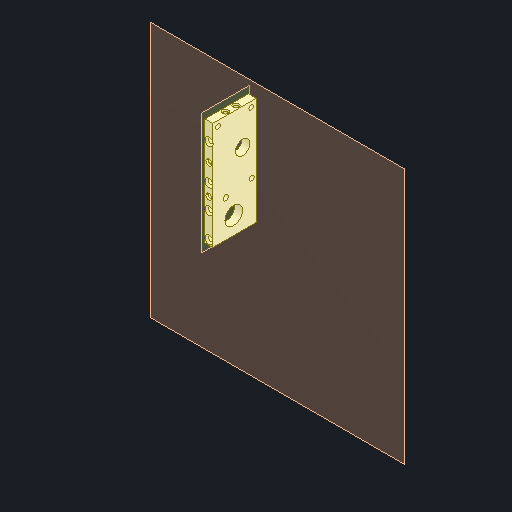
# Autodesk Inventor part: right_gear_holder
Saved by Autodesk Inventor 2023 (Build 270158000, 158)
## iProperties
Created: 2024-04-23
Part Number: right_gear_holder
Material: Nylon 6/6
Document SubType Name: Modeling
Designer: szymo
Density: 1.13 g/cm^3
Appearance: Nylon 6
Mass: 14.9327 g
Surface Area: 88.4291 cm^2
Volume: 13.2148 cm^3
Author: szymo
Autodesk Inventor part; units mm, degrees
ref_plane "YZ Plane" through (0, 0, 0) normal (1, 0, 0) x (0, 1, 0)
ref_plane "XZ Plane" through (0, 0, 0) normal (0, 1, 0) x (-1, 0, 0)
ref_plane "Work Plane1" through (0, 0, 0) normal (0, 0, 1) x (1, 0, 0)
sketch "Sketch1" plane through (0, 0, 0) normal (0, 0, 1) x (1, 0, 0)
  line L0 (23.5, 88.5) -> (-23.5, 88.5) projected
  line L1 (-23.5, 88.5) -> (-23.5, 36.5) projected
  line L2 (-26.5, 33.5) -> (-89, 33.5) projected
  line L3 (-89, 33.5) -> (-89, -72.5) projected
  line L4 (-89, -72.5) -> (-77, -72.5) projected
  line L5 (-74, -75.5) -> (-74, -93.5) projected
  line L6 (-74, -93.5) -> (74, -93.5) projected
  line L7 (74, -93.5) -> (74, -75.5) projected
  line L8 (77, -72.5) -> (89, -72.5) projected
  line L9 (89, -72.5) -> (89, 33.5) projected
  line L10 (89, 33.5) -> (26.5, 33.5) projected
  line L11 (23.5, 36.5) -> (23.5, 88.5) projected
  line L12 (-4.5, 81.5) -> (-4.5, 36.5) projected
  line L13 (-7.5, 33.5) -> (-13.5, 33.5) projected
  line L14 (-16.5, 36.5) -> (-16.5, 81.5) projected
  line L15 (7.5, 84.5) -> (13.5, 84.5) projected
  line L16 (16.5, 81.5) -> (16.5, 36.5) projected
  line L17 (13.5, 33.5) -> (7.5, 33.5) projected
  line L18 (4.5, 36.5) -> (4.5, 81.5) projected
  line L19 (-13.5, 84.5) -> (-7.5, 84.5) projected
  line L20 (-16.5, 88.5) -> (-22.5, 88.5)
  line L21 (-22.5, 88.5) -> (-22.5, 3.75)
  line L22 (-22.5, 3.75) -> (-16.5, 3.75)
  line L23 (-16.5, 3.75) -> (-16.5, 88.5)
  line L24 (-32.2, 4.75) -> (-59.9, 4.75)
  arc A0 (13.5, 33.5) -> (16.5, 36.5) centre (13.5, 36.5) ccw projected
  arc A1 (4.5, 36.5) -> (7.5, 33.5) centre (7.5, 36.5) ccw projected
  arc A2 (7.5, 84.5) -> (4.5, 81.5) centre (7.5, 81.5) ccw projected
  arc A3 (16.5, 81.5) -> (13.5, 84.5) centre (13.5, 81.5) ccw projected
  arc A4 (-4.5, 81.5) -> (-7.5, 84.5) centre (-7.5, 81.5) ccw projected
  arc A5 (-7.5, 33.5) -> (-4.5, 36.5) centre (-7.5, 36.5) ccw projected
  arc A6 (-16.5, 36.5) -> (-13.5, 33.5) centre (-13.5, 36.5) ccw projected
  arc A7 (-13.5, 84.5) -> (-16.5, 81.5) centre (-13.5, 81.5) ccw projected
  arc A8 (-26.5, 33.5) -> (-23.5, 36.5) centre (-26.5, 36.5) ccw projected
  arc A9 (-74, -75.5) -> (-77, -72.5) centre (-77, -75.5) ccw projected
  arc A10 (77, -72.5) -> (74, -75.5) centre (77, -75.5) ccw projected
  arc A11 (23.5, 36.5) -> (26.5, 33.5) centre (26.5, 36.5) ccw projected
  circle A12 centre (39.125, 25.9125) radius 1.0065 projected
  circle A13 centre (72.95, 12.275) radius 1.0065 projected
  circle A14 centre (-39.125, 12.3375) radius 1.0065 projected
  circle A15 centre (-72.95, 25.975) radius 1.0065 projected
  circle A16 centre (-72.95, 12.275) radius 1.0065 projected
  circle A17 centre (-39.125, 25.9125) radius 1.0065 projected
  circle A18 centre (72.95, 25.975) radius 1.0065 projected
  circle A19 centre (39.125, 12.3375) radius 1.0065 projected
  circle A20 centre (-42.4984, -44.6666) radius 1.2295 projected
  circle A21 centre (-79, -42.3889) radius 1.2295 projected
  circle A22 centre (-19.5, 28.875) radius 1.2295 projected
  circle A23 centre (19.5, 9.55) radius 1.2295 projected
  circle A24 centre (19.5, 47.3) radius 1.2295 projected
  circle A25 centre (-19.5, 47.3) radius 1.2295 projected
  circle A26 centre (0, 74.7) radius 1.2295 projected
  circle A27 centre (-19.4231, 74.8077) radius 1.2295 projected
  circle A28 centre (19.5, 74.7) radius 1.2295 projected
  circle A29 centre (0, 49.05) radius 1.2295 projected
  circle A30 centre (19.5, 28.875) radius 1.2295 projected
  circle A31 centre (0, 19.125) radius 1.2295 projected
  circle A32 centre (-19.5, 9.55) radius 1.2295 projected
  circle A33 centre (42.5, -44.6649) radius 1.2295 projected
  circle A34 centre (79, -42.3889) radius 1.2295 projected
  circle A35 centre (21.5, -85.5) radius 1.8 projected
  circle A36 centre (-64.5, -85.5) radius 1.8 projected
  circle A37 centre (-21.5, -85.5) radius 1.8 projected
  circle A38 centre (64.5, -85.5) radius 1.8 projected
  line L25 (-57, -78.5) -> (-82, -60.2553) projected
  line L26 (-82, -60.2553) -> (-82, -45.3889) projected
  line L27 (-76, -45.3889) -> (-45.4984, -47.6666) projected
  line L28 (-21.1, -27.9) -> (-21.1, -21.9) projected
  line L29 (-45.4984, -41.6666) -> (-76, -39.3889) projected
  line L30 (-82, -39.3889) -> (-82, 4.75) projected
  line L31 (30.3333, 4.75) -> (82, 4.75) projected
  line L32 (82, 4.75) -> (82, -39.3889) projected
  line L33 (76, -39.3889) -> (45.5, -41.6649) projected
  line L34 (21.1, -21.9) -> (21.1, -27.9) projected
  line L35 (45.5, -47.6649) -> (76, -45.3889) projected
  line L36 (82, -45.3889) -> (82, -60.2553) projected
  line L37 (82, -60.2553) -> (57, -78.5) projected
  line L38 (57, -78.5) -> (57, -87.5) projected
  arc A39 (55, -89.5) -> (57, -87.5) centre (55, -87.5) ccw projected
  line L39 (55, -89.5) -> (31, -89.5) projected
  arc A40 (29, -87.5) -> (31, -89.5) centre (31, -87.5) ccw projected
  line L40 (29, -87.5) -> (29, -78.5) projected
  line L41 (14, -78.5) -> (14, -87.5) projected
  arc A41 (12, -89.5) -> (14, -87.5) centre (12, -87.5) ccw projected
  line L42 (12, -89.5) -> (-12, -89.5) projected
  arc A42 (-14, -87.5) -> (-12, -89.5) centre (-12, -87.5) ccw projected
  line L43 (-14, -87.5) -> (-14, -78.5) projected
  line L44 (-29, -78.5) -> (-29, -87.5) projected
  arc A43 (-31, -89.5) -> (-29, -87.5) centre (-31, -87.5) ccw projected
  line L45 (-31, -89.5) -> (-55, -89.5) projected
  arc A44 (-57, -87.5) -> (-55, -89.5) centre (-55, -87.5) ccw projected
  line L46 (-57, -87.5) -> (-57, -78.5) projected
  line L47 (-69.95, 28.9125) -> (-42.125, 28.9125) projected
  line L48 (-42.125, 28.9125) -> (-42.125, 9.275) projected
  line L49 (-42.125, 9.275) -> (-69.95, 9.275) projected
  line L50 (-69.95, 9.275) -> (-69.95, 28.9125) projected
  line L51 (-16.5, 9.75) -> (-16.5, 28.5) projected
  line L52 (-16.5, 28.5) -> (-4.5, 28.5) projected
  line L53 (-4.5, 28.5) -> (-4.5, 9.75) projected
  line L54 (-4.5, 9.75) -> (-16.5, 9.75) projected
  line L55 (69.95, 9.3375) -> (42.125, 9.3375) projected
  line L56 (42.125, 9.3375) -> (42.125, 28.975) projected
  line L57 (42.125, 28.975) -> (69.95, 28.975) projected
  line L58 (69.95, 28.975) -> (69.95, 9.3375) projected
  line L59 (4.5, 9.75) -> (4.5, 28.5) projected
  line L60 (4.5, 28.5) -> (16.5, 28.5) projected
  line L61 (16.5, 28.5) -> (16.5, 9.75) projected
  line L62 (16.5, 9.75) -> (4.5, 9.75) projected
  line L63 (45.5, -41.6649) -> (27.1, -21.9) projected
  line L64 (27.1, -21.9) -> (30.3333, 4.75) projected
  line L65 (-45.4984, -47.6666) -> (-29, -78.5) projected
  line L66 (-82, 4.75) -> (-30.3333, 4.75) projected
  line L67 (-30.3333, 4.75) -> (-27.1, -21.9) projected
  line L68 (-27.1, -21.9) -> (-45.4984, -41.6666) projected
  line L69 (29, -78.5) -> (45.5, -47.6649) projected
  line L70 (-14, -78.5) -> (-39, -45.3279) projected
  line L71 (-39, -44.2124) -> (-21.1, -27.9) projected
  line L72 (-21.1, -21.9) -> (-24.3333, 4.75) projected
  line L73 (-24.3333, 4.75) -> (24.3333, 4.75) projected
  line L74 (24.3333, 4.75) -> (21.1, -21.9) projected
  line L75 (21.1, -27.9) -> (39.5, -44.6649) projected
  line L76 (39.5, -44.6649) -> (14, -78.5) projected
  circle A45 centre (-78, -67.1725) radius 1.2295 projected
  circle A46 centre (78, -67.1725) radius 1.2295 projected
  line L77 (-22.5, 28.9125) -> (-22.5, 9.55) projected
  line L78 (-22.5, 9.55) -> (-36.125, 9.55) projected
  line L79 (-36.125, 9.55) -> (-36.125, 28.9125) projected
  line L80 (-36.125, 28.9125) -> (-22.5, 28.9125) projected
  line L81 (76, -45.3889) -> (82, -45.3889) projected
  line L82 (82, -39.3889) -> (76, -39.3889) projected
  line L83 (36.125, 9.275) -> (22.5, 9.275) projected
  line L84 (22.5, 9.275) -> (22.5, 28.9125) projected
  line L85 (22.5, 28.9125) -> (36.125, 28.9125) projected
  line L86 (36.125, 28.9125) -> (36.125, 9.275) projected
  line L87 (-86, 28.975) -> (-75.95, 28.975) projected
  line L88 (-75.95, 28.975) -> (-75.95, 9.275) projected
  line L89 (-75.95, 9.275) -> (-86, 9.275) projected
  line L90 (-86, 9.275) -> (-86, 28.975) projected
  line L91 (-82, -45.3889) -> (-76, -45.3889) projected
  line L92 (-76, -39.3889) -> (-82, -39.3889) projected
  line L93 (75.95, 28.975) -> (86, 28.975) projected
  line L94 (86, 28.975) -> (86, 9.275) projected
  line L95 (86, 9.275) -> (75.95, 9.275) projected
  line L96 (75.95, 9.275) -> (75.95, 28.975) projected
  line L97 (-39, -45.3279) -> (-39, -44.2124) projected
  circle A47 centre (-24.1, -73.1) radius 1.2295 projected
  circle A48 centre (24.1, -24.9) radius 1.2295 projected
  circle A49 centre (-24.1, -24.9) radius 1.2295 projected
  circle A50 centre (24.1, -73.1) radius 1.2295 projected
  point P0 (0, 0)
  point P1 (-16.5, 36.5)
  point P2 (-16.5, 81.5)
  point P3 (7.5, 81.5)
  point P4 (13.5, 81.5)
  point P5 (-7.5, 81.5)
  point P6 (-13.5, 81.5)
  point P7 (-77, -75.5)
  point P8 (39, -44.2094)
  point P9 (-79, -67.8878)
  point P10 (-79, -66.4572)
  point P11 (-22.5, 25.9125)
  point P12 (-22.5, 12.55)
  point P13 (7.5, 81.5)
  point P14 (13.5, 81.5)
  point P15 (-7.5, 81.5)
  point P16 (-13.5, 81.5)
  dimension "d0" = 1
  dimension "d2" = 1
  constraints: 10 end point, 2 horizontal, 2 parallel, 1 collinear, 1 perpendicular, 1 point on line, 2 other
  measures "d0" distance between parallel lines of L1 L21
  measures "d2" distance between parallel lines of L24 L22
ref_plane "Work Plane2" through (-89, -40.3889, 33.5) normal (0, 0, 1) x (1, 0, 0)
extrude "Extrusion1" add sketch "Sketch1" along normal up to surface (33.5 mm away) contours L23 L14 L73 L21 L0 | L73 L23 L22 L21 | A22 | A25 | A27 | A32
sketch "Sketch2" plane through (-22.5, 3.75, 0) normal (-1, 0, 0) x (0, 0, 1)
  arc A0 (15.7043, 9.7757) -> (16.863, 11.545) centre (12.3771, 13.2188) ccw projected
  arc A1 (16.863, 11.545) -> (17.4685, 11.512) centre (17.375, 15.375) ccw projected
  arc A2 (17.4685, 11.512) -> (18.4285, 9.6275) centre (22.1095, 12.6893) ccw projected
  arc A3 (18.4285, 9.6275) -> (19.3146, 9.863) centre (17.375, 15.375) ccw projected
  arc A4 (19.3146, 9.863) -> (19.2121, 11.9755) centre (14.599, 10.6929) ccw projected
  arc A5 (19.2121, 11.9755) -> (19.7212, 12.3047) centre (17.375, 15.375) ccw projected
  arc A6 (19.7212, 12.3047) -> (21.6056, 11.3444) centre (22.7839, 15.9851) ccw projected
  arc A7 (21.6056, 11.3444) -> (22.184, 12.0558) centre (17.375, 15.375) ccw projected
  arc A8 (22.184, 12.0558) -> (20.8594, 13.7045) centre (17.8813, 9.9554) ccw projected
  arc A9 (20.8594, 13.7045) -> (21.0778, 14.2702) centre (17.375, 15.375) ccw projected
  arc A10 (21.0778, 14.2702) -> (23.1668, 14.6008) centre (21.3923, 19.0479) ccw projected
  arc A11 (23.1668, 14.6008) -> (23.2166, 15.5164) centre (17.375, 15.375) ccw projected
  arc A12 (23.2166, 15.5164) -> (21.1758, 16.0716) centre (20.9701, 11.288) ccw projected
  arc A13 (21.1758, 16.0716) -> (21.02, 16.6576) centre (17.375, 15.375) ccw projected
  arc A14 (21.02, 16.6576) -> (22.5157, 18.153) centre (18.4662, 20.7077) ccw projected
  arc A15 (22.5157, 18.153) -> (22.0178, 18.923) centre (17.375, 15.375) ccw projected
  arc A16 (22.0178, 18.923) -> (20.0404, 18.1726) centre (22.6858, 14.1817) ccw projected
  arc A17 (20.0404, 18.1726) -> (19.57, 18.5552) centre (17.375, 15.375) ccw projected
  arc A18 (19.57, 18.5552) -> (19.9011, 20.644) centre (15.1233, 20.3306) ccw projected
  arc A19 (19.9011, 20.644) -> (19.0457, 20.9743) centre (17.375, 15.375) ccw projected
  arc A20 (19.0457, 20.9743) -> (17.887, 19.205) centre (22.3729, 17.5312) ccw projected
  arc A21 (17.887, 19.205) -> (17.2815, 19.238) centre (17.375, 15.375) ccw projected
  arc A22 (17.2815, 19.238) -> (16.3215, 21.1225) centre (12.6405, 18.0607) ccw projected
  arc A23 (16.3215, 21.1225) -> (15.4354, 20.887) centre (17.375, 15.375) ccw projected
  arc A24 (15.4354, 20.887) -> (15.5379, 18.7745) centre (20.151, 20.0571) ccw projected
  arc A25 (15.5379, 18.7745) -> (15.0288, 18.4453) centre (17.375, 15.375) ccw projected
  arc A26 (15.0288, 18.4453) -> (13.1444, 19.4056) centre (11.9661, 14.7649) ccw projected
  arc A27 (13.1444, 19.4056) -> (12.566, 18.6942) centre (17.375, 15.375) ccw projected
  arc A28 (12.566, 18.6942) -> (13.8906, 17.0455) centre (16.8687, 20.7946) ccw projected
  arc A29 (13.8906, 17.0455) -> (13.6722, 16.4798) centre (17.375, 15.375) ccw projected
  arc A30 (13.6722, 16.4798) -> (11.5832, 16.1492) centre (13.3577, 11.7021) ccw projected
  arc A31 (11.5832, 16.1492) -> (11.5334, 15.2336) centre (17.375, 15.375) ccw projected
  arc A32 (11.5334, 15.2336) -> (13.5742, 14.6784) centre (13.7799, 19.462) ccw projected
  arc A33 (13.5742, 14.6784) -> (13.73, 14.0924) centre (17.375, 15.375) ccw projected
  arc A34 (13.73, 14.0924) -> (12.2343, 12.597) centre (16.2838, 10.0423) ccw projected
  arc A35 (12.2343, 12.597) -> (12.7322, 11.827) centre (17.375, 15.375) ccw projected
  arc A36 (12.7322, 11.827) -> (14.7096, 12.5774) centre (12.0642, 16.5683) ccw projected
  arc A37 (14.7096, 12.5774) -> (15.18, 12.1948) centre (17.375, 15.375) ccw projected
  arc A38 (15.18, 12.1948) -> (14.8489, 10.106) centre (19.6267, 10.4194) ccw projected
  arc A39 (14.8489, 10.106) -> (15.7043, 9.7757) centre (17.375, 15.375) ccw projected
  circle A40 centre (17.375, 15.375) radius 6.75
  circle A41 centre (17.375, 15.375) radius 5.8433
  line L0 (23.2183, 15.375) -> (24.125, 15.375)
  circle A42 centre (10.5, 57.25) radius 5.5 projected
  point P0 (0, -3.75)
  dimension "d6" = 13.5
  dimension "d5" = 0.9067
  dimension "d9" = 11
  constraints: 3 horizontal, 2 coincident, 2 end point, 2 horizontal alignment, 5 other
  measures "d5" distance of L0.start L0.end
  measures "d9" diameter of A42
extrude "Extrusion2" cut sketch "Sketch2" against normal up to next contours A39 A38 A37 A36 A35 A34 A33 A32 A31 A30 A29 A28 A27 A26 A25 A24 A23 A22 A21 A20 A19 A18 A17 A16 A15 A14 A13 A12 A11 A10 A9 A8 A7 A6 A5 A4 A3 A2 A1 A0 | A0 A1 A2 A41 | A41 A36 A37 A38 | A4 A5 A6 A41 | A41 A32 A33 A34 | A8 A9 A10 A41 | A41 A28 A29 A30 | A41 A24 A25 A26 | A12 A13 A14 A41 | A41 A20 A21 A22 | A16 A17 A18 A41 | A40 | A42
sketch "Sketch3" plane through (-16.5, 3.75, 0) normal (1, 0, 0) x (0, 0, -1)
  circle A0 centre (-23.4363, 30.1825) radius 2 projected
  point P0 (0, -3.75)
extrude "Extrusion3" cut sketch "Sketch3" against normal blind 5
ref_plane "Work Plane3" through (-23.5, 3.75, 0) normal (-1, 0, 0) x (0, 0, 1)
sketch "Sketch5" plane through (-23.5, 3.75, 0) normal (-1, 0, 0) x (0, 0, 1)
  circle A0 centre (29.5, 80.75) radius 2.1 projected
  circle A1 centre (4, 80.75) radius 2.1 projected
  circle A2 centre (3.5, 33.25) radius 2.1 projected
  point P0 (0, -3.75)
hole "Hole1" at (-23.5, 84.5, 29.5) at (-23.5, 84.5, 4) at (-23.5, 37, 3.5) direction (1, 0, 0) diameter 3.6 end through all countersink diameter 6.2 countersink angle 90 clearance for "Countersunk Flat Head Screw ISO 2009/7046" size "M3" standard "ISO"
sketch "Sketch6" plane through (-22.5, 3.75, 33.5) normal (0, 0, 1) x (1, 0, 0)
  line L0 (0, 8.625) -> (0, 22.125) projected
  line L1 (1, 32.1825) -> (1, 28.1825) projected
  line L2 (0, 31.15) -> (0, 35.35) projected
  line L3 (0, 51.75) -> (0, 62.75) projected
  line L4 (0, 78.65) -> (0, 82.85) projected
  line L5 (0, 78.65) -> (0, 82.85) projected
  line L6 (6, 0) -> (0, 0) projected
  line L7 (6, 84.75) -> (6, 0) projected
  line L8 (0, 84.75) -> (6, 84.75) projected
  line L9 (0, 0) -> (0, 84.75) projected
  line L10 (6, 28.125) -> (0, 28.125)
  line L11 (0, 28.125) -> (0, 35.35)
  line L12 (0, 35.35) -> (6, 35.35)
  line L13 (6, 35.35) -> (6, 28.125)
  line L14 (0, 8.625) -> (6, 8.625) projected
  line L15 (6, 8.625) -> (0, 8.625)
  line L16 (0, 8.625) -> (0, 22.125)
  line L17 (0, 22.125) -> (6, 22.125)
  line L18 (6, 22.125) -> (6, 8.625)
  line L19 (6, 78.95) -> (0.3, 78.95) projected
  line L20 (6, 84.75) -> (0, 84.75) projected
  line L21 (6, 78.95) -> (0, 78.95)
  line L22 (0, 78.95) -> (0, 84.75)
  line L23 (0, 84.75) -> (6, 84.75)
  line L24 (6, 84.75) -> (6, 78.95)
  line L25 (0, 51.75) -> (6, 51.75) projected
  line L26 (0, 51.75) -> (0, 62.75) projected
  line L27 (6, 51.75) -> (0, 51.75)
  line L28 (0, 51.75) -> (0, 62.75)
  line L29 (0, 62.75) -> (6, 62.75)
  line L30 (6, 62.75) -> (6, 51.75)
  line L31 (6, 0) -> (0, 0)
  line L32 (0, 0) -> (0, 4)
  line L33 (0, 4) -> (6, 4)
  line L34 (6, 4) -> (6, 0)
  circle A0 centre (3, 5.8) radius 1.8
  line L35 (6, 22.125) -> (0, 28.125)
  line L36 (0, 22.125) -> (6, 28.125)
  line L37 (6, 35.35) -> (0, 51.75)
  line L38 (0, 35.35) -> (6, 51.75)
  line L39 (0.3, 82.55) -> (0.3, 78.95) projected
  line L40 (6, 62.75) -> (0.3, 78.95)
  line L41 (6, 82.55) -> (6, 78.95) projected
  line L42 (0.3, 78.95) -> (6, 78.95)
  line L43 (6, 78.95) -> (0, 62.75)
  point P0 (22.5, -3.75)
  point P1 (3, 25.125)
  point P2 (3.0769, 71.0577)
  point P3 (3, 43.55)
  dimension "d20" = 4
  dimension "d21" = 3.6
  dimension "d22" = 3
  dimension "d23" = 3
  constraints: 54 end point, 10 parallel, 7 perpendicular, 6 point on line, 5 horizontal, 2 midpoint, 1 centre point, 1 coincident, 1 tangent, 5 other
  measures "d20" distance of L31.end L32.end
  measures "d21" diameter of A0
  measures "d23" distance from line of A0.centre L9
hole "Hole2" at (-19.5, 28.875, 33.5) at (-19.5, 9.55, 33.5) at (-19.4231, 74.8077, 33.5) at (-19.5, 47.3, 33.5) direction (0, 0, -1) diameter 3.6 end through all countersink diameter 6.3 countersink angle 90 clearance for "Countersunk Flat Head Screw ISO 2009/7046" size "M3" standard "ISO"
sketch "Sketch9" plane through (-22.5, 88.5, 0) normal (0, 1, 0) x (1, 0, 0)
  circle A0 centre (22.5, -20.825) radius 2.3 projected
  circle A1 centre (22.5, -12.675) radius 2.3 projected
  line L0 (18, -33.5) -> (27, -33.5) projected
  line L1 (27, 0) -> (27, -33.5) projected
  line L2 (27, 0) -> (18, 0) projected
  line L3 (18, 0) -> (18, -33.5) projected
  line L4 (22.5, -20.825) -> (0, -20.825)
  line L5 (0, -24.125) -> (0, -10.625) projected
  line L6 (22.5, -12.675) -> (0, -12.675)
  line L7 (6, 0) -> (6, -33.5) projected
  point P0 (22.5, 0)
  point P1 (3, -20.825)
  point P2 (3, -12.675)
  dimension "d45" = 3
  dimension "d46" = 3
  dimension "d47" = 3
  dimension "d48" = 3
  constraints: 4 end point, 4 point on line, 1 horizontal, 1 perpendicular
  measures "d45" distance from line of point (3, -20.825) L5
  measures "d46" distance from line of L7 point (3, -20.825)
  measures "d47" distance from line of L7 point (3, -12.675)
  measures "d48" distance from line of point (3, -12.675) L5
hole "Hole5" at (-19.5, 88.5, 20.825) at (-19.5, 88.5, 12.675) direction (0, -1, 0) diameter 4 depth 6 counterbore diameter 4.6 counterbore depth 1.5
sketch "Sketch10" plane through (-19.5, 47.3, 33.5) normal (0, 0, 1) x (1, 0, 0)
  line L0 (-3, 8.2) -> (-3, 19.2) projected
  arc A0 (3, -17.4645) -> (-3, -17.4645) centre (0, -18.425) ccw projected
  arc A1 (-3, -0.9605) -> (3, -0.9605) centre (0, 0) ccw projected
  arc A2 (3, -17.4645) -> (-3, -17.4645) centre (0, -18.425) ccw projected
  line L1 (3, -0.9605) -> (3, -17.4645) projected
  arc A3 (-3, -0.9605) -> (3, -0.9605) centre (0, 0) ccw projected
  line L2 (-3, -17.4645) -> (-3, -0.9605) projected
  line L3 (3, 8.2) -> (-3, 8.2)
  line L4 (3, 19.2) -> (-3, 19.2)
  line L5 (-3, 19.2) -> (3, 8.2)
  line L6 (-3, 8.2) -> (3, 19.2)
  line L7 (3, -17.4645) -> (-3, -0.9605)
  line L8 (-3, -17.4645) -> (3, -0.9605)
  point P0 (19.5, -47.3)
  point P1 (0, -9.2125)
  point P2 (0, 13.7)
  constraints: 12 end point, 2 horizontal, 2 midpoint, 2 other
hole "Hole6" at (-19.5, 38.0875, 33.5) at (-19.5, 61, 33.5) direction (0, 0, -1) diameter 4 depth 6 counterbore diameter 4.6 counterbore depth 1.5
sketch "Sketch11" plane through (-22.5, 3.75, 0) normal (0, -1, 0) x (1, 0, 0)
  line L0 (6, 33.5) -> (0, 33.5) projected
  line L1 (0, 0) -> (0, 33.5) projected
  line L2 (0, 0) -> (6, 0) projected
  line L3 (6, 0) -> (6, 33.5) projected
  point P0 (22.5, 0)
extrude "Extrusion4" cut sketch "Sketch11" against normal blind 2
equation "\"d22\" = d23"
equation "\"d45\" = d46"
equation "\"d47\" = d48"
body "Solid1"
